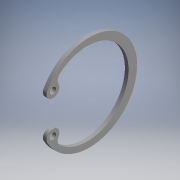
# Autodesk Inventor part: RRING-C-INT-S-37
Saved by Autodesk Inventor 2017.3 (Build 213256000, 256)
## iProperties
Part Number: RRING-C-INT-S-37
Material: Generic
Catalog Web Link: www.cadenas.de
Description: RRING_C_INT-Retaining Rings - C  (Internal)
Vendor: MISUMI
Document SubType Name: Modeling
Designer: partserver
Manufacturer: MISUMI
Mass: 0.442654 g
Surface Area: 9.28198 cm^2
Volume: 0.442654 cm^3
Density: 1 g/cm^3
Appearance: PSOLRGB-192-192-192
Category: PARTsolutions
Company: MISUMI
Title: RRING-C-INT-S-37
Author: Cadenas PARTsolutions
Comments: Retaining Rings - C  (Internal)
PSOL_IDENT_0: {$CADENAS_DATA\23d-libs\misumi\metric\accessories\rring_c_int.prj},181 {VTYP=3D},{NB=RRING-C-INT-S-3
PSOL_IDENT_1: 7},{LINA=RRING-C-INT-S-37},{NN=RRING_C_INT},{DATE=30.10.2020 15:47:10},{GEOMDATE=05.03.2015 00:00:00
PSOL_IDENT_2: },{VERSION=},{LINEID=330},{WBVAR=MAT},{WBNUMERIC=}  {NB=RRING-C-INT-S-37},{LINA=RRING-C-INT-S-37},{K
PSOL_IDENT_3: T=DUMMY},{PN=RRING-C-INT-S-37},{TYPE=RRING-C-INT},{MAT=-S},{HARD=36~44HRC},{NO=37},{DD3=39.8},{DD3TO
PSOL_IDENT_4: L=+0.25/-0.25},{TT=1.50},{TTTOL=+0.06/-0.06},{BB=3.5},{AA=5.2},{DD0=2.5},{DD4=26},{DD1=37},{DD2=39.0
PSOL_IDENT_5: },{DD2TOL=+0.25/0},{MM=1.75},{MMTOL=+0.14/0},{NN=2.0},{A2=16.10}
NB: RRING-C-INT-S-37
NN: 2
NT: Retaining Rings - C  (Internal)
NBSYN: $PN.
LINA: RRING-C-INT-S-37
CATALOG: Misumi
PN: RRING-C-INT-S-37
MAT: 304 Stainless Steel-CSP
HARD: 36~44HRC
NO: 37
DD3: 39.8
DD3TOL: +0.25/-0.25
TT: 1.5
TTTOL: +0.06/-0.06
BB: 3.5
AA: 5.2
DD0: 2.5
DD4: 26
DD1: 37
DD2: 39
DD2TOL: +0.25/0
MM: 1.75
MMTOL: +0.14/0
SUPPLIER: MISUMI
ARTICLENO: RRING-C-INT-S-37
BOMINFO: RRING-C-INT-S-37
CREATOR: CADENAS GmbH
Autodesk Inventor part; units mm, degrees
ref_plane "YZ Plane" through (0, 0, 0) normal (1, 0, 0) x (0, 1, 0)
ref_plane "XZ Plane" through (0, 0, 0) normal (0, 1, 0) x (-1, 0, 0)
ref_plane "XY Plane" through (0, 0, 0) normal (0, 0, 1) x (1, 0, 0)
sketch "Sketch_3" plane through (0, 0, 0) normal (1, 0, 0) x (0, 1, 0)
  arc A0 (-17.209, -9.1705) -> (-17.209, 9.1705) centre (0, 0) ccw
  arc A1 (-17.209, 9.1705) -> (-15.8412, 5.6396) centre (-15.0028, 7.9948) ccw
  line L0 (-15.8412, 5.6396) -> (-15.7316, 5.6006)
  arc A2 (-15.7316, 5.6006) -> (-12.612, 9.3571) centre (-14.8596, 8.05) ccw
  arc A3 (-12.0929, 12.6065) -> (-12.612, 9.3571) centre (-10.3645, 10.6642) ccw
  arc A4 (-12.0929, -12.6065) -> (-12.0929, 12.6065) centre (-0.875, 0) ccw
  arc A5 (-12.612, -9.3571) -> (-12.0929, -12.6065) centre (-10.3645, -10.6642) ccw
  arc A6 (-12.612, -9.3571) -> (-15.7316, -5.6006) centre (-14.8596, -8.05) ccw
  line L1 (-15.7316, -5.6006) -> (-15.8412, -5.6396)
  arc A7 (-15.8412, -5.6396) -> (-17.209, -9.1705) centre (-15.0028, -7.9948) ccw
  circle A8 centre (-14.8596, -8.05) radius 1.25
  circle A9 centre (-14.8596, 8.05) radius 1.25
  constraints: 16 point on circle, 10 centre point, 4 end point
extrude "Extrusion1" add sketch "Sketch_3" along normal mid plane 1.5
ref_plane "rr_XY" through (-0.75, 0, 0) normal (1, 0, 0) x (0, 0, -1)
ref_plane "rr_YZ" through (-0.75, 0, 0) normal (0, 0, -1) x (0, 1, 0)
ref_plane "rr_ZX" through (-0.75, 0, 0) normal (0, 1, 0) x (1, 0, 0)
body "Solid1"
